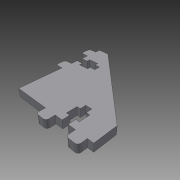
# Autodesk Inventor part: y_motor_mount_brace
Saved by Autodesk Inventor 2014 (Build 180170000, 170)
## iProperties
Created: 2013-12-07
Part Number: y_motor_mount_brace
Material: Generic
Document SubType Name: Modeling
Designer: buben
Density: 1 g/cm^3
Appearance: Default
Author: buben
Autodesk Inventor part; units mm, degrees
ref_plane "YZ Plane" through (0, 0, 0) normal (1, 0, 0) x (0, 1, 0)
ref_plane "XZ Plane" through (0, 0, 0) normal (0, 1, 0) x (-1, 0, 0)
ref_plane "XY Plane" through (0, 0, 0) normal (0, 0, 1) x (1, 0, 0)
sketch "Sketch1" plane through (0, 0, 0) normal (0, 0, 1) x (1, 0, 0)
  line L0 (0, 67.3) -> (0, 0)
  line L1 (0, 0) -> (60, 0)
  line L2 (60, 0) -> (60, 16)
  line L3 (60, 16) -> (8, 67.3)
  line L4 (8, 67.3) -> (0, 67.3)
  dimension "d0" = 67.3
  dimension "d1" = 8
  dimension "d2" = 16
  dimension "d3" = 60
  constraints: 10 end point, 2 parallel, 1 perpendicular, 1 vertical
  measures "d0" distance of L0.start L0.end
  measures "d1" distance of L3.end L0.start
  measures "d2" distance of L1.end L2.end
  measures "d3" distance of L0.end L1.end
extrude "Extrusion1" add sketch "Sketch1" along normal blind 6
sketch "Sketch2" plane through (0, 0, 6) normal (0, 0, 1) x (1, 0, 0)
  line L0 (0, 67.3) -> (0, 0) projected
  line L1 (0, 0) -> (60, 0) projected
  line L2 (60, 0) -> (60, 16) projected
  line L3 (8, 67.3) -> (0, 67.3) projected
  line L4 (16.3, 50.05) -> (16.3, 45.55)
  line L5 (0, 45.55) -> (0, 50.05)
  line L6 (5, 52.55) -> (12.3, 52.55)
  line L7 (12.3, 43.05) -> (5, 43.05)
  line L8 (38.25, 16.3) -> (42.75, 16.3)
  line L9 (42.75, 0) -> (38.25, 0)
  line L10 (45.25, 12.3) -> (45.25, 5)
  line L11 (35.75, 5) -> (35.75, 12.3)
  line L12 (5, 43.05) -> (5, 45.55)
  line L13 (5, 50.05) -> (5, 52.55)
  line L14 (12.3, 52.55) -> (12.3, 50.05)
  line L15 (12.3, 45.55) -> (12.3, 43.05)
  line L16 (0, 50.05) -> (5, 50.05)
  line L17 (12.3, 50.05) -> (16.3, 50.05)
  line L18 (16.3, 45.55) -> (12.3, 45.55)
  line L19 (5, 45.55) -> (0, 45.55)
  line L20 (35.75, 12.3) -> (38.25, 12.3)
  line L21 (42.75, 12.3) -> (45.25, 12.3)
  line L22 (45.25, 5) -> (42.75, 5)
  line L23 (38.25, 5) -> (35.75, 5)
  line L24 (38.25, 0) -> (38.25, 5)
  line L25 (38.25, 12.3) -> (38.25, 16.3)
  line L26 (42.75, 16.3) -> (42.75, 12.3)
  line L27 (42.75, 5) -> (42.75, 0)
  point P0 (16.3, 47.8)
  point P1 (40.5, 16.3)
  dimension "d6" = 4.5
  dimension "d7" = 5
  dimension "d8" = 7.3
  dimension "d9" = 4
  dimension "d10" = 2.5
  dimension "d11" = 19.5
  dimension "d12" = 19.5
  constraints: 48 end point, 20 parallel, 10 collinear, 8 perpendicular, 7 equal length, 6 horizontal, 2 midpoint
  measures "d6" distance of L4.start L4.end
  measures "d7" distance of L5.end L13.start
  measures "d8" distance of L6.start L6.end
  measures "d9" distance of L14.end L4.start
  measures "d10" distance of L13.start L6.start
  measures "d11" distance from line of point (16.3, 47.8) L3
  measures "d12" distance from line of L2 point (40.5, 16.3)
extrude "Extrusion2" cut sketch "Sketch2" against normal blind 6
sketch "Sketch3" plane through (0, 0, 6) normal (0, 0, 1) x (1, 0, 0)
  line L0 (0, 45.55) -> (0, 0) projected
  line L1 (0, 0) -> (38.25, 0) projected
  line L2 (38.25, 16.3) -> (42.75, 16.3) projected
  line L3 (42.75, 0) -> (60, 0) projected
  line L4 (0, 67.3) -> (0, 50.05) projected
  line L5 (16.3, 50.05) -> (16.3, 45.55) projected
  line L6 (0, 40.3) -> (-4, 40.3)
  line L7 (-6, 38.3) -> (-6, 34.3)
  line L8 (-4, 32.3) -> (0, 32.3)
  line L9 (0, 32.3) -> (0, 40.3)
  line L10 (0, 63.3) -> (-4, 63.3)
  line L11 (-6, 61.3) -> (-6, 57.3)
  line L12 (-4, 55.3) -> (0, 55.3)
  line L13 (0, 55.3) -> (0, 63.3)
  line L14 (25, 0) -> (33, 0)
  line L15 (33, 0) -> (33, -4)
  line L16 (31, -6) -> (27, -6)
  line L17 (25, -4) -> (25, 0)
  line L18 (48, 0) -> (56, 0)
  line L19 (56, 0) -> (56, -4)
  line L20 (54, -6) -> (50, -6)
  line L21 (48, -4) -> (48, 0)
  arc A0 (-4, 63.3) -> (-6, 61.3) centre (-4, 61.3) ccw
  arc A1 (-6, 57.3) -> (-4, 55.3) centre (-4, 57.3) ccw
  arc A2 (-4, 40.3) -> (-6, 38.3) centre (-4, 38.3) ccw
  arc A3 (-6, 34.3) -> (-4, 32.3) centre (-4, 34.3) ccw
  arc A4 (25, -4) -> (27, -6) centre (27, -4) ccw
  arc A5 (31, -6) -> (33, -4) centre (31, -4) ccw
  arc A6 (48, -4) -> (50, -6) centre (50, -4) ccw
  arc A7 (54, -6) -> (56, -4) centre (54, -4) ccw
  point P0 (16.3, 47.8)
  point P1 (40.5, 16.3)
  dimension "d15" = 2
  dimension "d16" = 8
  dimension "d17" = 8
  dimension "d18" = 8
  dimension "d19" = 8
  dimension "d20" = 6
  dimension "d21" = 6
  dimension "d22" = 15
  dimension "d23" = 15
  dimension "d24" = 7.5
  dimension "d25" = 7.5
  constraints: 32 end point, 16 point on circle, 16 tangent, 8 centre point, 8 parallel, 7 equal radius, 4 horizontal, 4 perpendicular, 4 point on line, 2 collinear, 2 midpoint
  measures "d15" radius of A0
  measures "d16" distance between parallel lines of L12 L10
  measures "d17" distance between parallel lines of L8 L6
  measures "d18" distance between parallel lines of L15 L17
  measures "d19" distance between parallel lines of L19 L21
  measures "d20" distance between parallel lines of L4 L11
  measures "d21" distance between parallel lines of L1 L16
  measures "d22" distance between parallel lines of L6 L12
  measures "d23" distance between parallel lines of L21 L15
  measures "d24" distance from line of L12 point (16.3, 47.8)
  measures "d25" distance from line of L15 point (40.5, 16.3)
extrude "Extrusion3" add sketch "Sketch3" against normal blind 6
body "Solid1"
